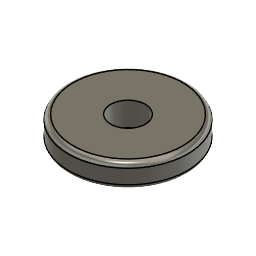
MurlokVR_M1.4_Washers_v1.0 (Autodesk Fusion 360 design; units mm, degrees)
part number: 2026-06-28-14-49-14-930
Autodesk Fusion 360 part; units mm, degrees
sketch "Sketch1" plane through (0, 0, 0) normal (0, 1, 0) x (1, 0, 0)
  circle A0 centre (0, 0) radius 0.725
  circle A1 centre (0, 0) radius 2.5
  dimension "d1" = 1.45
  dimension "d2" = 5
  constraint coincident A0.centre A1.centre
  constraint concentric A0 A1
  measures "d1" diameter of A0
  measures "d2" diameter of A1
extrude "Extrude1" add sketch "Sketch1" along normal blind 1
fillet "Fillet1" radius 0.2 2 edges at (-2.3308, 1, 0.904) (-2.3308, 0, 0.904)
